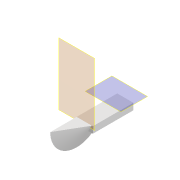
# Autodesk Inventor part: encoder guard
Saved by Autodesk Inventor 2020 (Build 240168000, 168)
## iProperties
Created: 2020-01-15
Part Number: encoder guard
Material: Generic
Document SubType Name: Modeling
Designer: ball
Density: 1 g/cm^3
Appearance: Default
Author: ball
Autodesk Inventor part; units mm, degrees
ref_plane "YZ Plane" through (0, 0, 0) normal (1, 0, 0) x (0, 1, 0)
ref_plane "XZ Plane" through (0, 0, 0) normal (0, 1, 0) x (-1, 0, 0)
ref_plane "XY Plane" through (0, 0, 0) normal (0, 0, 1) x (1, 0, 0)
ref_plane "Work Plane1" through (0, 0, 0) normal (0, 0, 1) x (1, 0, 0)
sketch "Sketch1" plane through (0, 0, 0) normal (0, 0, 1) x (1, 0, 0)
  line L0 (25.4, -44.45) -> (0, -44.45) construction
  line L1 (25.4, -44.45) -> (12.7, -44.45)
  line L2 (12.7, -65.151) -> (25.4, -44.45)
  line L3 (12.7, -44.45) -> (12.7, -65.151)
  point P0 (0, 0)
  dimension "d0" = 20.701
  dimension "d1" = 12.7
  constraints: 6 end point, 1 midpoint, 1 perpendicular, 1 point on line
  measures "d0" distance from line of L0 L2.start
  measures "d1" distance from line of L1.start L3
revolve "Revolution1" add sketch "Sketch1" angle 180 mid plane about axis through (25.4, -44.45, 0) along (-1, 0, 0)
ref_plane "Work Plane2" through (12.7, -44.45, -31.115) normal (0, -1, 0) x (0, 0, -1)
sketch "Sketch2" plane through (12.7, -44.45, -31.115) normal (0, -1, 0) x (0, 0, -1)
  line L0 (0.635, -12.7) -> (0.635, 12.7) construction
  line L1 (9.525, 12.7) -> (-9.525, 12.7) construction
  line L2 (0.635, 0) -> (-31.115, 0)
  line L3 (-31.115, 0) -> (-31.115, 12.7)
  line L4 (-31.115, 12.7) -> (0.635, 12.7)
  line L5 (0.635, 12.7) -> (0.635, 0)
  point P0 (-31.115, -12.7)
  constraints: 8 end point, 2 parallel, 1 horizontal, 1 midpoint, 1 perpendicular
extrude "Extrusion1" add sketch "Sketch2" along normal blind 5.08
body "Solid1"
